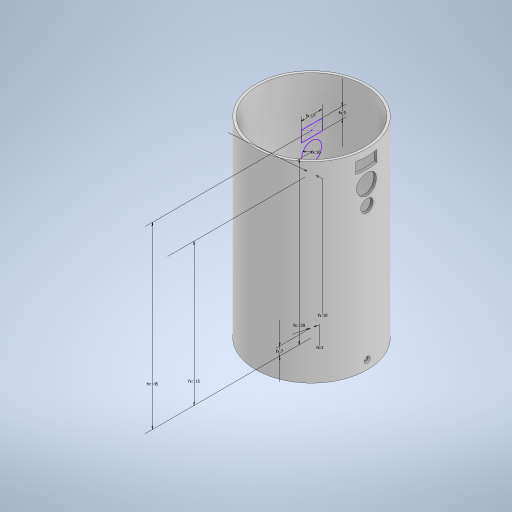
# Autodesk Inventor part: Vedro-Z_tube
Saved by Autodesk Inventor 2024 (Build 280153000, 153)
## iProperties
Created: 2024-02-28
Part Number: Vedro-Z_tube
Material: Generic
Document SubType Name: Modeling
Designer: Andrei
Density: 1 g/cm^3
Appearance: Default
Author: Andrei
Autodesk Inventor part; units mm, degrees
ref_plane "YZ Plane" through (0, 0, 0) normal (1, 0, 0) x (0, 1, 0)
ref_plane "XZ Plane" through (0, 0, 0) normal (0, 1, 0) x (-1, 0, 0)
ref_plane "XY Plane" through (0, 0, 0) normal (0, 0, 1) x (1, 0, 0)
sketch "Sketch1" plane through (0, 0, 0) normal (0, 1, 0) x (-1, 0, 0)
  circle A0 centre (0, 0) radius 45
  circle A1 centre (0, 0) radius 43
  dimension "d0" = 90
  dimension "d1" = 86
  constraints: 2 centre point, 2 coincident
  measures "d0" diameter of A0
  measures "d1" diameter of A1
sketch "Sketch2" plane through (0, 0, 0) normal (1, 0, 0) x (0, 1, 0)
  circle A0 centre (130, 0) radius 8
  circle A1 centre (115, 0) radius 5
  line L0 (149.5, 8.5) -> (140.5, 8.5)
  line L1 (140.5, 8.5) -> (140.5, -8.5)
  line L2 (140.5, -8.5) -> (149.5, -8.5)
  line L3 (149.5, -8.5) -> (149.5, 8.5)
  line L4 (149.5, 8.5) -> (140.5, -8.5) construction
  line L5 (140.5, 8.5) -> (149.5, -8.5) construction
  circle A2 centre (7, 0) radius 1.5
  point P0 (0, 0)
  point P1 (145, 0)
  dimension "d2" = 16
  dimension "d3" = 130
  dimension "d4" = 10
  dimension "d5" = 115
  dimension "d6" = 9
  dimension "d7" = 17
  dimension "d8" = 145
  dimension "d15" = 3
  dimension "d16" = 7
  constraints: 12 end point, 3 centre point, 2 midpoint, 2 parallel, 1 horizontal, 1 perpendicular
  measures "d2" diameter of A0
  measures "d3" distance of point (0, 0) A0.centre
  measures "d4" diameter of A1
  measures "d5" distance of point (0, 0) A1.centre
  measures "d6" distance of L2.end L1.end
  measures "d7" distance of L1.end L0.end
  measures "d8" distance of point (0, 0) point (145, 0)
  measures "d15" diameter of A2
  measures "d16" distance of A2.centre point (0, 0)
extrude "Extrusion1" add sketch "Sketch1" along normal blind 155
extrude "Extrusion2" cut sketch "Sketch2" along normal blind 155 contours A0 | A1 | L3 L2 L1 L0
extrude "Extrusion3" cut sketch "Sketch2" along normal mid plane 155 contours A2
chamfer "Chamfer1" distance 1 angle 45 3 edges at (-44.975, 6.9999, -1.5) (-44.975, 7.0001, 1.5) (45, 5.5, 0.0096)
chamfer_without_effect "Chamfer2"
equation "\"d0\" = dExternal"
equation "\"d1\" = dExternal - 2 * wWall"
equation "\"d2\" = dUSBHole"
equation "\"d4\" = dPowerHole"
equation "\"d6\" = zUSB"
equation "\"d7\" = wUSBHole"
equation "\"d15\" = dHoles"
equation "\"d16\" = hHoles"
equation "\"d9\" = hTube"
equation "\"d11\" = hTube"
equation "\"d17\" = hTube"
equation "\"dExternal\" = 90"
equation "\"wWall\" = 2"
equation "\"dUSBHole\" = 16"
equation "\"dPowerHole\" = 10"
equation "\"hUSBHole\" = 175"
equation "\"wUSBHole\" = 17"
equation "\"hDUSBHole\" = 145"
equation "\"hPowerHole\" = 175"
equation "\"zUSB\" = 9"
equation "\"hTube\" = 155"
equation "\"dHoles\" = 3"
equation "\"hHoles\" = 7"
body "Solid1"
